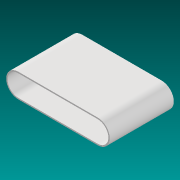
# Autodesk Inventor part: 皮带3
Saved by Autodesk Inventor 2021 (Build 250183000, 183)
## iProperties
Created: 2025-04-17
Part Number: 皮带3
Material: 常规
Document SubType Name: Modeling
Designer: 86155
Density: 1 g/cm^3
Appearance: 默认
Author: 86155
Autodesk Inventor part; units mm, degrees
ref_plane "YZ Plane" through (0, 0, 0) normal (1, 0, 0) x (0, 1, 0)
ref_plane "XZ Plane" through (0, 0, 0) normal (0, 1, 0) x (-1, 0, 0)
ref_plane "XY Plane" through (0, 0, 0) normal (0, 0, 1) x (1, 0, 0)
sketch "草图1" plane through (0, 0, 0) normal (0, 0, 1) x (1, 0, 0)
  arc A0 (0.1539, 22.4995) -> (0.7588, -22.4872) centre (0, 0) ccw
  arc A1 (298.5893, -12.4375) -> (297.0703, 32.5368) centre (297.8305, 10.0497) ccw
  line L0 (0.1539, 22.4995) -> (297.0703, 32.5368)
  line L1 (298.5893, -12.4375) -> (0.7588, -22.4872)
  line L2 (296.9014, 37.534) -> (0.0814, 27.4999)
  arc A2 (0.0814, 27.4999) -> (0.9274, -27.4844) centre (0, 0) ccw
  line L3 (0.9274, -27.4844) -> (298.7579, -17.4347)
  arc A3 (298.7579, -17.4347) -> (296.9014, 37.534) centre (297.8305, 10.0497) ccw
  dimension "d0" = 45
  dimension "d1" = 45
  dimension "d2" = 298
  dimension "d3" = 5
  constraints: 8 end point, 8 point on circle, 4 centre point, 3 tangent, 1 coincident, 3 other
  measures "d0" diameter of A0
  measures "d1" diameter of A1
  measures "d2" distance of A1.centre A0.centre
  measures "d3" distance between parallel lines of L0 L2
extrude "拉伸1" add sketch "草图1" along normal blind 240
